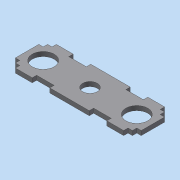
# Autodesk Inventor part: Bearing-Middle
Saved by Autodesk Inventor 2016 SP1 (Build 200210100, 210)
## iProperties
Created: 2016-03-01
Part Number: Bearing-Middle
Material: Generic
Document SubType Name: Modeling
Designer: Mohamed A.
Density: 1 g/cm^3
Appearance: Default
Author: Mohamed A.
Autodesk Inventor part; units mm, degrees
ref_plane "YZ Plane" through (0, 0, 0) normal (1, 0, 0) x (0, 1, 0)
ref_plane "XZ Plane" through (0, 0, 0) normal (0, 1, 0) x (-1, 0, 0)
ref_plane "XY Plane" through (0, 0, 0) normal (0, 0, 1) x (1, 0, 0)
sketch "Sketch2" plane through (0, 0, 0) normal (0, 0, 1) x (1, 0, 0)
  line L0 (-60.2, 0) -> (60.2, 0) construction
  line L1 (0, -19.6) -> (0, 19.6) construction
  circle A0 centre (0, 0) radius 5
  circle A1 centre (-32, 0) radius 7.5
  circle A2 centre (32, 0) radius 7.5
  line L2 (43, 11) -> (37, 11)
  line L3 (-43, 11) -> (-43, 8)
  line L4 (-43, -11) -> (-37, -11)
  line L5 (43, -11) -> (43, -8)
  line L6 (-43, 11) -> (-43, 14)
  line L7 (-43, 14) -> (-37, 14)
  line L8 (43, 14) -> (43, 11)
  line L9 (-43, -11) -> (-43, -14)
  line L10 (-43, -14) -> (-37, -14)
  line L11 (43, -14) -> (43, -11)
  line L12 (40, 11) -> (40, 8)
  line L13 (40, 8) -> (43, 8)
  line L14 (40, -8) -> (43, -8)
  line L15 (-40, 11) -> (-40, 8)
  line L16 (-40, 8) -> (-43, 8)
  line L17 (-40, -8) -> (-43, -8)
  line L18 (-40, 8) -> (-40, -11)
  line L19 (-43, 8) -> (-43, -11)
  line L20 (40, 8) -> (40, -11)
  line L21 (43, 8) -> (43, 11)
  line L22 (43, -8) -> (43, 8)
  line L23 (22.5, 14) -> (22.5, 11) construction
  line L24 (25.5, 14) -> (25.5, 11)
  line L25 (40, 11) -> (40, 14) construction
  line L26 (37, 14) -> (37, 11)
  line L27 (37, 14) -> (43, 14)
  line L28 (25.5, 14) -> (37, 14)
  line L29 (25.5, 11) -> (13.5, 11)
  line L30 (37, 11) -> (25.5, 11)
  line L31 (-25.5, 14) -> (-25.5, 11)
  line L32 (-37, 14) -> (-37, 11)
  line L33 (-25.5, 14) -> (-13.5, 14)
  line L34 (-37, 14) -> (-25.5, 14)
  line L35 (-37, 11) -> (-43, 11)
  line L36 (-25.5, 11) -> (-37, 11)
  line L37 (13.5, 14) -> (13.5, 11)
  line L38 (-13.5, 14) -> (-13.5, 11)
  line L39 (-13.5, 14) -> (25.5, 14)
  line L40 (-13.5, 11) -> (-25.5, 11)
  line L41 (13.5, 11) -> (-13.5, 11)
  line L42 (25.5, -14) -> (25.5, -11)
  line L43 (37, -14) -> (37, -11)
  line L44 (-25.5, -14) -> (-25.5, -11)
  line L45 (-37, -14) -> (-37, -11)
  line L46 (13.5, -14) -> (13.5, -11)
  line L47 (-13.5, -14) -> (-13.5, -11)
  line L48 (37, -11) -> (43, -11)
  line L49 (25.5, -11) -> (37, -11)
  line L50 (13.5, -11) -> (25.5, -11)
  line L51 (-13.5, -11) -> (13.5, -11)
  line L52 (-25.5, -11) -> (-13.5, -11)
  line L53 (-37, -11) -> (-25.5, -11)
  line L54 (-37, -14) -> (-25.5, -14)
  line L55 (-25.5, -14) -> (-13.5, -14)
  line L56 (-13.5, -14) -> (13.5, -14)
  line L57 (13.5, -14) -> (25.5, -14)
  line L58 (25.5, -14) -> (37, -14)
  line L59 (37, -14) -> (43, -14)
  dimension "d0" = 10
  dimension "d1" = 15
  dimension "d2" = 15
  dimension "d3" = 32
  dimension "d4" = 32
  dimension "d5" = 11
  dimension "d6" = 22
  dimension "d9" = 3
  dimension "d11" = 3
  dimension "d12" = 3
  dimension "d13" = 3
  dimension "d14" = 20.5
  dimension "d15" = 3
  dimension "d16" = 3
  dimension "d17" = 9
  dimension "d18" = 12
  constraints: 116 end point, 79 perpendicular, 57 parallel, 21 point on line, 16 symmetric about line, 7 horizontal, 5 midpoint, 5 vertical, 3 centre point, 1 coincident, 1 collinear, 3 other
  measures "d0" diameter of A0
  measures "d1" diameter of A1
  measures "d2" diameter of A2
  measures "d3" distance of A1.centre point (0, 0)
  measures "d4" distance of A2.centre point (0, 0)
  measures "d5" distance from line of A1.centre L3
  measures "d6" distance between parallel lines of L4 L2
  measures "d9" distance of L3.start L6.end
  measures "d11" distance between parallel lines of L5 L12
  measures "d12" distance between parallel lines of L13 L2
  measures "d13" distance between parallel lines of L3 L15
  measures "d14" distance between parallel lines of L22 L23
  measures "d15" distance between parallel lines of L23 L24
  measures "d16" distance between parallel lines of L26 L25
  measures "d17" distance between parallel lines of L37 L23
  measures "d18" distance between parallel lines of L31 L38
extrude "Extrusion1" add sketch "Sketch2" along normal mid plane 3 contours L12 L20 L48 L49 L50 L51 L52 L53 L4 L18 L15 L35 L36 L40 L41 L29 L30 L2 | L22 L14 L20 L13 | L30 L24 L28 L26 | L41 L38 L39 L37 | L43 L58 L42 L49 | L36 L32 L34 L31 | L46 L56 L47 L51 | L18 L17 L19 L16 | L44 L54 L45 L53
body "Solid1"
